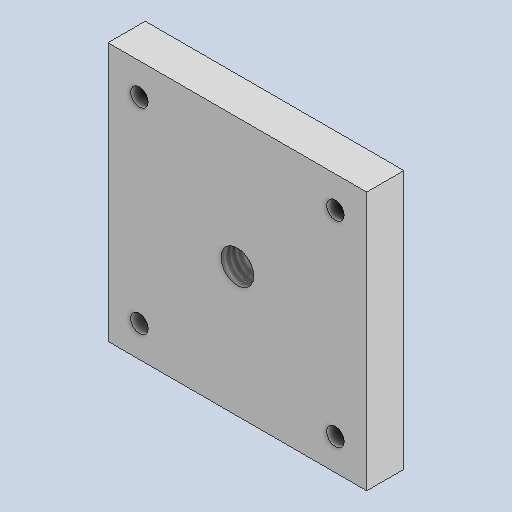
# Autodesk Inventor part: Acoplador do pé nivelador
Saved by Autodesk Inventor 2026 (Build 300175050, 175E)
## iProperties
Created: 2025-08-25
Part Number: Acoplador do pé nivelador
Material: Genérico
Document SubType Name: Modeling
Designer: Kedson Neves
Density: 1 g/cm^3
Appearance: Padrão
Description: Acoplador do pé nivelador
Author: Kedson Neves
Autodesk Inventor part; units mm, degrees
ref_plane "YZ Plane" through (0, 0, 0) normal (1, 0, 0) x (0, 1, 0)
ref_plane "XZ Plane" through (0, 0, 0) normal (0, 1, 0) x (-1, 0, 0)
ref_plane "XY Plane" through (0, 0, 0) normal (0, 0, 1) x (1, 0, 0)
sketch "Esboço1" plane through (0, 0, 0) normal (0, 0, 1) x (1, 0, 0)
  circle A0 centre (-25.0665, 24.8448) radius 1.621
  circle A1 centre (24.9335, -25.1552) radius 1.621
  line L0 (-25.0665, 24.8448) -> (24.9335, -25.1552)
  line L1 (-33.0665, -33.1552) -> (32.9335, -33.1552)
  line L2 (32.9335, -33.1552) -> (32.9335, 32.8448)
  line L3 (32.9335, 32.8448) -> (-33.0665, 32.8448)
  line L4 (-33.0665, 32.8448) -> (-33.0665, -33.1552)
  line L5 (-33.0665, -33.1552) -> (32.9335, 32.8448) construction
  line L6 (32.9335, -33.1552) -> (-33.0665, 32.8448) construction
  circle A2 centre (-0.0665, -0.1552) radius 2.5192
  circle A3 centre (24.9335, 24.8448) radius 1.621
  circle A4 centre (-25.0665, -25.1552) radius 1.621
  point P0 (0, 0)
  dimension "d0" = 66
  dimension "d1" = 66
  constraints: 14 end point, 5 centre point, 3 midpoint, 2 parallel, 1 coincident, 1 horizontal, 1 perpendicular
  measures "d0" distance of L2.end L3.end
  measures "d1" distance of L3.end L1.start
extrude "Extrusão1" add sketch "Esboço1" along normal blind 9.5
sketch "Esboço2" plane through (0, 0, 9.5) normal (0, 0, 1) x (1, 0, 0)
  circle A0 centre (24.9335, 24.8448) radius 1.621 projected
  circle A1 centre (-25.0665, 24.8448) radius 1.621 projected
  circle A2 centre (-25.0665, -25.1552) radius 1.621 projected
  circle A3 centre (24.9335, -25.1552) radius 1.621 projected
  point P0 (0, 0)
  constraints: 4 coincident
hole "Furo1" at (24.9335, 24.8448, 9.5) at (-25.0665, 24.8448, 9.5) at (-25.0665, -25.1552, 9.5) at (24.9335, -25.1552, 9.5) direction (0, 0, -1) diameter 4.5 end through all clearance for "Countersunk Flat Head Screw ISO 2009/7046" size "M4" standard "ISO"
sketch "Esboço3" plane through (0, 0, 9.5) normal (0, 0, 1) x (1, 0, 0)
  circle A0 centre (-0.0665, -0.1552) radius 2.5192 projected
  point P0 (0, 0)
  constraints: 1 coincident
hole "Furo2" at (-0.0665, -0.1552, 9.5) direction (0, 0, -1) diameter 8.376 end through all thread size "M10x1.5" class "6H" standard "ISO Metric profile"
